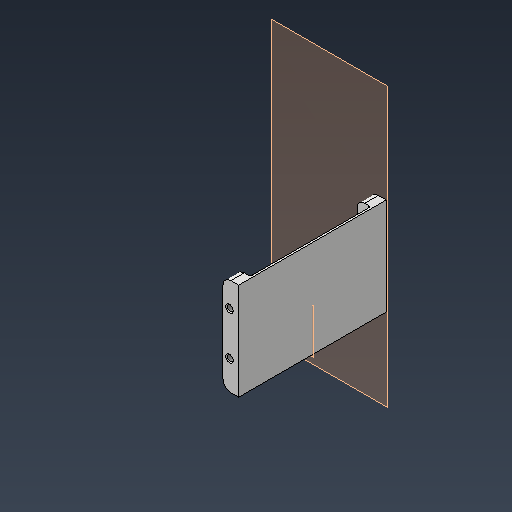
# Autodesk Inventor part: DriverDownholdAlternate
Saved by Autodesk Inventor 2026.2 (Build 302298010, 298A)
## iProperties
Created: 2026-07-05
Part Number: DriverDownholdAlternate
Material: Generic
Document SubType Name: Modeling
Designer: szymo
Density: 1 g/cm^3
Appearance: Default
Author: szymo
Autodesk Inventor part; units mm, degrees
note: some values were not read from the file. Chosen so that the rebuilt part matches the saved one: edges of "Fillet2".
ref_plane "YZ Plane" through (0, 0, 0) normal (1, 0, 0) x (0, 1, 0)
ref_plane "XZ Plane" through (0, 0, 0) normal (0, 1, 0) x (-1, 0, 0)
ref_plane "XY Plane" through (0, 0, 0) normal (0, 0, 1) x (1, 0, 0)
ref_plane "Work Plane1" through (0, 0, 0) normal (0, 0, 1) x (1, 0, 0)
sketch "Sketch1" plane through (0, 0, 0) normal (0, 0, 1) x (1, 0, 0)
  circle A0 centre (23.85, -37.9212) radius 0.7 projected
  circle A1 centre (23.85, -26.8413) radius 0.7 projected
  circle A2 centre (10.55, -52.3871) radius 14 projected
  circle A3 centre (10.55, -11.45) radius 14 projected
  line L0 (25.25, -34.8579) -> (25.25, -62.5871) projected
  line L1 (22.15, -44.5487) -> (26.25, -44.5487)
  line L2 (26.25, -44.5487) -> (26.25, -19.2884)
  line L3 (26.25, -19.2884) -> (22.15, -19.2884)
  line L4 (22.15, -19.2884) -> (22.15, -44.5487)
  circle A4 centre (24.2, -42.4987) radius 2.05
  circle A5 centre (24.2, -21.3384) radius 2.05
  point P0 (0, 0)
  point P1 (24.2, -19.2884)
  point P2 (22.15, -21.3384)
  point P3 (22.15, -42.4987)
  point P4 (24.2, -44.5487)
  dimension "d0" = 1
  dimension "d1" = 1
  constraints: 8 end point, 6 tangent, 2 centre point, 2 parallel, 1 horizontal, 1 perpendicular, 4 other
  measures "d0" distance between parallel lines of L2 L0
  measures "d1" distance edge to line of A0 L4
extrude "Extrusion1" add sketch "Sketch1" along normal blind 3.5 contours A0 | A1 | A4 L0 L1 | A4 L0 | L4 A5 L2 A4 | L0 A4 L2 L1 | L0 A4 | A5 | L3 L2 A5
sketch "Sketch2" plane through (0, 0, 3.5) normal (0, 0, 1) x (1, 0, 0)
  line L0 (22.25, -33.4185) -> (19.55, -33.4185) projected
  line L1 (22.25, -30.4185) -> (19.55, -30.4185) projected
  line L2 (26.25, -33.9066) -> (26.25, -41.9871) projected
  line L3 (26.25, -29.1685) -> (26.25, -34.6685) projected
  line L4 (26.25, -21.85) -> (26.25, -29.9304) projected
  line L5 (22.15, -21.3384) -> (22.15, -42.4987) projected
  line L6 (26.25, -33.9185) -> (20.65, -33.9185)
  line L7 (20.65, -33.9185) -> (20.65, -29.9185)
  line L8 (20.65, -29.9185) -> (26.25, -29.9185)
  line L9 (26.25, -29.9185) -> (26.25, -33.9185)
  point P0 (0, 0)
  dimension "d4" = 0.5
  dimension "d5" = 0.5
  dimension "d6" = 1.5
  constraints: 8 end point, 2 parallel, 1 horizontal, 1 perpendicular, 1 point on line
  measures "d4" distance between parallel lines of L0 L6
  measures "d5" distance between parallel lines of L8 L1
  measures "d6" distance between parallel lines of L7 L5
extrude "Extrusion2" add sketch "Sketch2" along normal blind 5.5
sketch "Sketch3" plane through (20.65, -33.9185, 3.5) normal (0, -1, 0) x (1, 0, 0)
  circle A0 centre (-2.1, 3) radius 1.25 projected
  line L0 (5.6, 0) -> (5.6, 5.5) projected
  circle A1 centre (2.4, 3) radius 1.25
  line L1 (2.4, 3) -> (-2.1, 3)
  circle A2 centre (2.4, 3) radius 2.5
  point P0 (-20.65, -3.5)
  dimension "d17" = 5
  dimension "d18" = 0.7
  constraints: 2 centre point, 2 end point, 1 coincident, 1 equal radius, 1 horizontal
  measures "d17" diameter of A2
  measures "d18" distance edge to line of A2 L0
extrude "Extrusion3" cut sketch "Sketch3" against normal blind 11.5 contours A1
fillet "Fillet1" radius 2 2 edges at (20.65, -31.9185, 9) (20.65, -31.9185, 3.5)
ref_plane "Work Plane2" through (0, 0, 19.2) normal (0, 0, 1) x (1, 0, 0)
mirror "Mirror1" about plane through (0, 0, 19.2) normal (0, 0, 1) of "Extrusion1", "Extrusion2", "Extrusion3", "Fillet1"
sketch "Sketch4" plane through (0, 0, 3.5) normal (0, 0, 1) x (1, 0, 0)
  line L0 (26.25, -44.5487) -> (26.25, -19.2884) projected
  line L1 (24.2, -44.5487) -> (26.25, -44.5487) projected
  line L2 (26.25, -19.2884) -> (24.2, -19.2884) projected
  line L3 (25.75, -44.5487) -> (25.75, -19.2884)
  arc A0 (22.15, -42.4987) -> (24.2, -44.5487) centre (24.2, -42.4987) ccw projected
  line L4 (22.15, -21.3384) -> (22.15, -42.4987) projected
  arc A1 (24.2, -19.2884) -> (22.15, -21.3384) centre (24.2, -21.3384) ccw projected
  line L5 (25.75, -40.5487) -> (22.15, -40.5487)
  point P0 (0, 0)
  dimension "d14" = 0.5
  dimension "d20" = 4
  constraints: 4 end point, 4 point on line, 2 perpendicular
  measures "d14" distance between parallel lines of L3 L0
  measures "d20" distance from line of L3.start L5
extrude "Extrusion4" add sketch "Sketch4" along normal up to surface (31.4 mm away) contours L1 L3 L2 L0 | L1 A0 L4 L5 L3
fillet "Fillet2" radius 0.5 7 edges at (25.75, -37.2336, 3.5) (25.75, -24.6035, 3.5) (25.75, -37.2336, 34.9) (25.75, -24.6035, 34.9) (25.75, -40.5487, 19.2) (25.75, -31.9185, 9) (25.75, -31.9185, 29.4)
sketch "Sketch5" plane through (24.2, -19.2884, 38.4) normal (0, 0, 1) x (1, 0, 0)
  circle A0 centre (-0.35, -17.7307) radius 0.7 projected
  circle A1 centre (-0.35, -6.4868) radius 0.7 projected
  point P0 (-24.2, 19.2884)
hole "Hole1" at (23.85, -37.0191, 38.4) at (23.85, -25.7752, 38.4) direction (0, 0, -1) diameter 1.567 depth 6.3 countersink diameter 2 countersink angle 90 thread size "M2x0.4" class "6H" standard "ISO Metric profile"
sketch "Sketch6" plane through (0, 0, 0) normal (0, 0, -1) x (-1, 0, 0)
  circle A0 centre (-23.85, -26.8413) radius 0.7 projected
  circle A1 centre (-23.85, -37.9212) radius 0.7 projected
  point P0 (0, 0)
hole "Hole2" at (23.85, -26.8413, 0) at (23.85, -37.9212, 0) direction (0, 0, 1) diameter 1.567 depth 6.3 countersink diameter 2 countersink angle 90 thread size "M2x0.4" class "6H" standard "ISO Metric profile"
equation "\"d5\" = d4"
body "Solid1"
